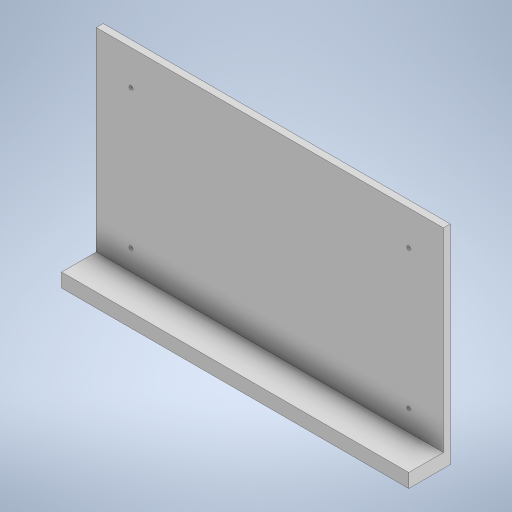
# Autodesk Inventor part: Part1
Saved by Autodesk Inventor 2024 (Build 280153000, 153)
## iProperties
Created: 2023-07-07
Part Number: Part1
Material: Generic
Document SubType Name: Modeling
Designer: ardab
Density: 1 g/cm^3
Appearance: Default
Author: ardab
Autodesk Inventor part; units mm, degrees
ref_plane "YZ Plane" through (0, 0, 0) normal (1, 0, 0) x (0, 1, 0)
ref_plane "XZ Plane" through (0, 0, 0) normal (0, 1, 0) x (-1, 0, 0)
ref_plane "XY Plane" through (0, 0, 0) normal (0, 0, 1) x (1, 0, 0)
sketch "Sketch1" plane through (0, 0, 0) normal (0, 0, 1) x (1, 0, 0)
  line L0 (250, -150) -> (-250, -150)
  line L1 (-250, -150) -> (-250, 150)
  line L2 (-250, 150) -> (250, 150)
  line L3 (250, 150) -> (250, -150)
  line L4 (250, -150) -> (-250, 150) construction
  line L5 (-250, -150) -> (250, 150) construction
  point P0 (0, 0)
  dimension "d0" = 500
  dimension "d1" = 300
  constraints: 12 end point, 2 midpoint, 2 parallel, 1 horizontal, 1 perpendicular
  measures "d0" distance of L1.end L2.end
  measures "d1" distance of L0.end L1.end
extrude "Extrusion1" add sketch "Sketch1" along normal blind 10
sketch "Sketch2" plane through (0, 0, 10) normal (0, 0, 1) x (1, 0, 0)
  line L0 (-250, 150) -> (-250, -150) projected
  line L1 (-250, -150) -> (250, -150) projected
  line L2 (-250, -130) -> (250, -130)
  line L3 (250, -130) -> (250, -150)
  line L4 (250, -150) -> (-250, -150)
  line L5 (-250, -150) -> (-250, -130)
  point P0 (0, 0)
  dimension "d6" = 20
  constraints: 8 end point, 2 parallel, 1 horizontal, 1 perpendicular, 1 point on line
  measures "d6" distance between parallel lines of L1 L2
extrude "Extrusion2" add sketch "Sketch2" along normal blind 50
sketch "Sketch3" plane through (0, 0, 0) normal (0, 0, -1) x (-1, 0, 0)
  line L0 (-250, -150) -> (-250, 150) projected
  line L1 (-250, 150) -> (250, 150) projected
  line L2 (250, 150) -> (250, -150) projected
  line L3 (250, -150) -> (-250, -150) projected
  point P0 (0, 0)
  point P1 (-200, 100)
  point P2 (200, 100)
  point P3 (-200, -100)
  point P4 (200, -100)
  dimension "d7" = 50
  dimension "d8" = 50
  dimension "d9" = 50
  dimension "d10" = 50
  dimension "d11" = 50
  dimension "d12" = 50
  dimension "d13" = 50
  dimension "d14" = 50
  measures "d7" distance from line of L0 point (-200, 100)
  measures "d8" distance from line of L1 point (-200, 100)
  measures "d9" distance from line of L1 point (200, 100)
  measures "d10" distance from line of L2 point (200, 100)
  measures "d11" distance from line of L2 point (200, -100)
  measures "d12" distance from line of L3 point (200, -100)
  measures "d13" distance from line of L3 point (-200, -100)
  measures "d14" distance from line of L0 point (-200, -100)
hole "Hole1" at (200, 100, 0) at (-200, 100, 0) at (200, -100, 0) at (-200, -100, 0) direction (0, 0, 1) diameter 5 end through all
body "Solid1"
